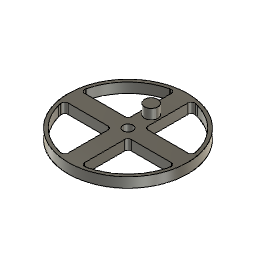
spinning_part_36mm_diameter v2 (Autodesk Fusion 360 design; units mm, degrees)
Autodesk Fusion 360 part; units mm, degrees
sketch "Sketch1" plane through (0, 0, 0) normal (0, 0, 1) x (1, 0, 0)
  circle A0 centre (0, 0) radius 18
  line L0 (-2.5, 3.5) -> (-2.5, 15.5984)
  line L1 (2.5, 15.5848) -> (2.5, 3.5)
  line L2 (3.5, 2.5) -> (15.5763, 2.5)
  line L3 (17.3145, 2.5) -> (17.3145, -2.5)
  line L4 (15.5763, -2.5) -> (3.5, -2.5)
  line L5 (-3.5, -2.5) -> (-15.5736, -2.5)
  line L6 (-15.5966, 2.5) -> (-3.5, 2.5)
  line L7 (2.5, -3.5) -> (2.5, -15.5822)
  line L8 (-2.5, -15.565) -> (-2.5, -3.5)
  arc A1 (3.5, -2.5) -> (2.5, -3.5) centre (3.5, -3.5) ccw
  arc A2 (-2.5, -3.5) -> (-3.5, -2.5) centre (-3.5, -3.5) ccw
  arc A3 (2.5, 3.5) -> (3.5, 2.5) centre (3.5, 3.5) ccw
  arc A4 (-3.5, 2.5) -> (-2.5, 3.5) centre (-3.5, 3.5) ccw
  line L9 (3.7044, 16.5636) -> (4.4389, 16.4103)
  line L10 (-3.6937, 16.5794) -> (-4.0793, 16.5033)
  arc A5 (-2.5, 15.5984) -> (-3.6937, 16.5794) centre (-3.5, 15.5984) ccw
  arc A6 (3.7044, 16.5636) -> (2.5, 15.5848) centre (3.5, 15.5848) ccw
  line L11 (16.5538, 3.711) -> (16.3494, 4.6582)
  line L12 (16.5538, -3.711) -> (16.3494, -4.6582)
  arc A7 (15.5763, 2.5) -> (16.5538, 3.711) centre (15.5763, 3.5) ccw
  arc A8 (16.5538, -3.711) -> (15.5763, -2.5) centre (15.5763, -3.5) ccw
  line L13 (3.7064, -16.5606) -> (4.506, -16.3919)
  line L14 (-3.7196, -16.5406) -> (-4.9466, -16.2644)
  arc A9 (-3.7196, -16.5406) -> (-2.5, -15.565) centre (-3.5, -15.565) ccw
  arc A10 (2.5, -15.5822) -> (3.7064, -16.5606) centre (3.5, -15.5822) ccw
  line L15 (-16.5774, 3.6951) -> (-16.4916, 4.1264)
  line L16 (-16.5507, -3.713) -> (-16.3296, -4.7268)
  arc A11 (-16.5774, 3.6951) -> (-15.5966, 2.5) centre (-15.5966, 3.5) ccw
  arc A12 (-15.5736, -2.5) -> (-16.5507, -3.713) centre (-15.5736, -3.5) ccw
  arc A13 (-16.3296, -4.7268) -> (-4.9466, -16.2644) centre (0, 0) ccw
  arc A14 (4.506, -16.3919) -> (16.3494, -4.6582) centre (0, 0) ccw
  arc A15 (16.3494, 4.6582) -> (4.4389, 16.4103) centre (0, 0) ccw
  arc A16 (-4.0793, 16.5033) -> (-16.4916, 4.1264) centre (0, 0) ccw
  circle A17 centre (0, 0) radius 1.5
  dimension "d1" = 34
  dimension "d2" = 36
  dimension "d7" = 1
  dimension "d8" = 1
  dimension "d9" = 1
  dimension "d10" = 1
  dimension "d11" = 1
  dimension "d12" = 1
  dimension "d13" = 1
  dimension "d14" = 1
  dimension "d15" = 1
  dimension "d16" = 1
  dimension "d17" = 1
  dimension "d18" = 1
  dimension "d19" = 3
  constraint vertical L0
  constraint vertical L1
  constraint horizontal L2
  constraint vertical L3
  constraint horizontal L4
  constraint horizontal L5
  constraint horizontal L6
  constraint vertical L7
  constraint vertical L8
  constraint tangent L7 A1
  constraint tangent L4 A1
  constraint tangent L5 A2
  constraint tangent L8 A2
  constraint tangent L1 A3
  constraint tangent L2 A3
  constraint tangent L6 A4
  constraint tangent L0 A4
  constraint coincident L9.end A13
  constraint coincident L10.end A13
  constraint tangent L10 A5
  constraint tangent L0 A5
  constraint tangent L9 A6
  constraint tangent L1 A6
  constraint coincident L11.end A13
  constraint coincident L12.end A13
  constraint coincident L3.start L2
  constraint tangent L11 A7
  constraint tangent L2 A7
  constraint coincident L3.end L4
  constraint tangent L4 A8
  constraint tangent L12 A8
  constraint coincident L13.end A13
  constraint tangent L14 A9
  constraint tangent L8 A9
  constraint tangent L13 A10
  constraint tangent L7 A10
  constraint tangent L15 A11
  constraint tangent L6 A11
  constraint tangent L16 A12
  constraint tangent L5 A12
  constraint concentric A13 A14
  constraint concentric A14 A15
  constraint concentric A15 A16
  constraint concentric A14 A17
  measures "d1" diameter of A13
  measures "d2" diameter of A0
  measures "d7" radius of A1
  measures "d8" radius of A2
  measures "d9" radius of A3
  measures "d10" radius of A4
  measures "d11" radius of A5
  measures "d12" radius of A6
  measures "d13" radius of A7
  measures "d14" radius of A8
  measures "d15" radius of A9
  measures "d16" radius of A10
  measures "d17" radius of A11
  measures "d18" radius of A12
  measures "d19" diameter of A17
extrude "Extrude1" add sketch "Sketch1" along normal blind 3
sketch "Sketch2" plane through (0, 0, 3) normal (0, 0, 1) x (-1, 0, 0)
  arc A0 (-16.5538, 3.711) -> (-15.5763, 2.5) centre (-15.5763, 3.5) ccw
  line L0 (-16.5538, 3.711) -> (-16.3494, 4.6582)
  arc A1 (-4.506, 16.3919) -> (-16.3494, 4.6582) centre (0, 0) ccw
  line L1 (-4.506, 16.3919) -> (-3.7064, 16.5606)
  arc A2 (-2.5, 15.5822) -> (-3.7064, 16.5606) centre (-3.5, 15.5822) ccw
  line L2 (-2.5, 15.5822) -> (-2.5, 3.5)
  arc A3 (-3.5, 2.5) -> (-2.5, 3.5) centre (-3.5, 3.5) ccw
  line L3 (-3.5, 2.5) -> (-15.5763, 2.5)
  circle A4 centre (0, 0) radius 1.5
  arc A5 (16.5774, -3.6951) -> (15.5966, -2.5) centre (15.5966, -3.5) ccw
  line L4 (16.5774, -3.6951) -> (16.4916, -4.1264)
  arc A6 (4.0793, -16.5033) -> (16.4916, -4.1264) centre (0, 0) ccw
  line L5 (4.0793, -16.5033) -> (3.6937, -16.5794)
  arc A7 (2.5, -15.5984) -> (3.6937, -16.5794) centre (3.5, -15.5984) ccw
  line L6 (2.5, -15.5984) -> (2.5, -3.5)
  arc A8 (3.5, -2.5) -> (2.5, -3.5) centre (3.5, -3.5) ccw
  line L7 (3.5, -2.5) -> (15.5966, -2.5)
  arc A9 (-3.7044, -16.5636) -> (-2.5, -15.5848) centre (-3.5, -15.5848) ccw
  line L8 (-3.7044, -16.5636) -> (-4.4389, -16.4103)
  arc A10 (-16.3494, -4.6582) -> (-4.4389, -16.4103) centre (0, 0) ccw
  line L9 (-16.3494, -4.6582) -> (-16.5538, -3.711)
  arc A11 (-15.5763, -2.5) -> (-16.5538, -3.711) centre (-15.5763, -3.5) ccw
  line L10 (-15.5763, -2.5) -> (-3.5, -2.5)
  arc A12 (-2.5, -3.5) -> (-3.5, -2.5) centre (-3.5, -3.5) ccw
  line L11 (-2.5, -3.5) -> (-2.5, -15.5848)
  arc A13 (3.7196, 16.5406) -> (2.5, 15.565) centre (3.5, 15.565) ccw
  line L12 (3.7196, 16.5406) -> (4.9466, 16.2644)
  arc A14 (16.3296, 4.7268) -> (4.9466, 16.2644) centre (0, 0) ccw
  line L13 (16.3296, 4.7268) -> (16.5507, 3.713)
  arc A15 (15.5736, 2.5) -> (16.5507, 3.713) centre (15.5736, 3.5) ccw
  line L14 (15.5736, 2.5) -> (3.5, 2.5)
  arc A16 (2.5, 3.5) -> (3.5, 2.5) centre (3.5, 3.5) ccw
  line L15 (2.5, 3.5) -> (2.5, 15.565)
  circle A17 centre (0, 0) radius 18
  circle A18 centre (0, -7) radius 2
  dimension "d23" = 4
  measures "d23" diameter of A18
extrude "Extrude2" add sketch "Sketch2" along normal blind 3 contours A18
